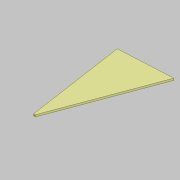
# Autodesk Inventor part: Pieskovy_luc
Saved by Autodesk Inventor 2018.1 (Build 221171000, 171)
## iProperties
Created: 2018-06-12
Part Number: Pieskovy_luc
Material: Všeobecné
Document SubType Name: Modeling
Designer: PS
Density: 1 g/cm^3
Appearance: Výchozí
Author: PS
Autodesk Inventor part; units mm, degrees
ref_plane "YZ Plane" through (0, 0, 0) normal (1, 0, 0) x (0, 1, 0)
ref_plane "XZ Plane" through (0, 0, 0) normal (0, 1, 0) x (-1, 0, 0)
ref_plane "XY Plane" through (0, 0, 0) normal (0, 0, 1) x (1, 0, 0)
sketch "Náčrt6" plane through (0, 0, 0) normal (0, 0, 1) x (1, 0, 0)
  line L0 (0, 10) -> (1200, 331.539)
  line L1 (0, 10) -> (0, 0)
  line L2 (0, -10) -> (1200, -331.539)
  line L3 (1200, 331.539) -> (1200, 0)
  line L4 (0, 0) -> (1200, 0) construction
  line L5 (1200, 0) -> (1200, -331.539)
  line L6 (0, 0) -> (0, -10)
  dimension "d15" = 20
  dimension "d16" = 30
  dimension "d17" = 1200
  constraints: 14 end point, 4 vertical, 1 collinear, 1 horizontal, 1 other
  measures "d15" distance of L2.start L0.start
  measures "d16" angle of L2 L0
  measures "d17" distance between parallel lines of L5 L1
extrude "Vysunutí3" add sketch "Náčrt6" along normal mid plane 20
sketch "Náčrt7" plane through (0, -10, 10) normal (-1, 0, 0) x (0, 0, 1)
  circle A0 centre (-10, 10) radius 5
  dimension "d22" = 10
  constraints: 1 centre point, 1 coincident
  measures "d22" diameter of A0
extrude "Vysunutí4" cut sketch "Náčrt7" against normal blind 20
